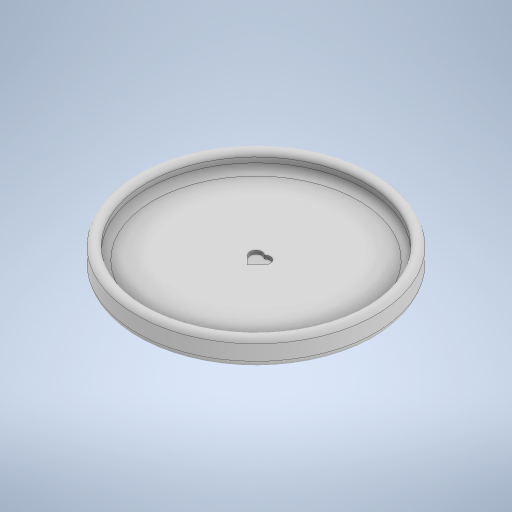
# Autodesk Inventor part: Orchid Coaster V3
Saved by Autodesk Inventor 2024 (Build 280153000, 153)
## iProperties
Created: 2024-02-28
Part Number: Orchid Coaster V3
Material: Generic
Document SubType Name: Modeling
Designer: haque
Density: 1 g/cm^3
Appearance: Default
Author: haque
Autodesk Inventor part; units mm, degrees
ref_plane "YZ Plane" through (0, 0, 0) normal (1, 0, 0) x (0, 1, 0)
ref_plane "XZ Plane" through (0, 0, 0) normal (0, 1, 0) x (-1, 0, 0)
ref_plane "XY Plane" through (0, 0, 0) normal (0, 0, 1) x (1, 0, 0)
sketch "Sketch1" plane through (0, 0, 0) normal (0, 1, 0) x (-1, 0, 0)
  circle A0 centre (0, 0) radius 32.5
  circle A1 centre (0, 0) radius 35.5
  dimension "d0" = 65
  dimension "d1" = 71
  constraints: 2 centre point, 2 coincident
  measures "d0" diameter of A0
  measures "d1" diameter of A1
extrude "Extrusion1" add sketch "Sketch1" along normal blind 8
extrude "Extrusion2" add sketch "Sketch1" along normal blind 3 contours A0
fillet "Fillet1" radius 2 2 edges at (35.5, 0, 0) (32.5, 3, 0)
fillet "Fillet2" radius 1.5 2 edges at (32.5, 8, 0) (35.5, 8, 0)
sketch "Sketch2" plane through (0, 3, 0) normal (0, 1, 0) x (1, 0, 0)
  line L0 (-2.5, -2.5) -> (2.5, -2.5)
  line L1 (2.5, -2.5) -> (2.5, 2.5)
  line L2 (2.5, 2.5) -> (-2.5, 2.5)
  line L3 (-2.5, 2.5) -> (-2.5, -2.5)
  line L4 (-2.5, -2.5) -> (2.5, 2.5) construction
  line L5 (2.5, -2.5) -> (-2.5, 2.5) construction
  line L6 (0, -2.5) -> (2.5, 0)
  line L7 (0, -2.5) -> (-2.5, 0)
  circle A0 centre (1.25, 1.25) radius 1.7678
  circle A1 centre (-1.25, 1.25) radius 1.7678
  point P0 (0, 0)
  point P1 (0, 2.5)
  dimension "d8" = 5
  dimension "d9" = 5
  constraints: 16 end point, 5 midpoint, 2 parallel, 2 point on line, 1 horizontal, 1 perpendicular, 6 other
  measures "d8" distance of L2.end L1.end
  measures "d9" distance of L1.end L0.end
extrude "Extrusion3" cut sketch "Sketch2" against normal blind 1 contours L7 A1 A0 L6 | A1 L3 | L3 L2 A0 A1 | A0 A1 L2 L1 | L1 A0 | A1 L2 | A0 A1 | L2 A0
body "Solid1"
